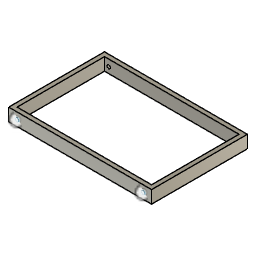
Power Supply Jig v4 (Autodesk Fusion 360 design; units mm, degrees)
Autodesk Fusion 360 part; units mm, degrees
sketch "jig" plane through (0, 0, 0) normal (0, 0, 1) x (1, 0, 0)
  line L0 (-150, 0) -> (20, 0)
  line L1 (-150, 0) -> (-150, 116)
  line L2 (-150, 116) -> (20, 116)
  line L3 (20, 116) -> (20, 0)
  line L4 (-144.988, 5.0299) -> (15.012, 5.0299)
  line L5 (-144.988, 5.0299) -> (-144.988, 111.0299)
  line L6 (15.012, 5.0299) -> (15.012, 111.0299)
  line L7 (15.012, 111.0299) -> (-144.988, 111.0299)
  dimension "d1" = 170
  dimension "d2" = 116
  dimension "d3" = 170
  dimension "d4" = 160
  dimension "d5" = 106
  dimension "d6" = 106
  constraint horizontal L0
  constraint perpendicular L0 L1
  constraint perpendicular L1 L2
  constraint perpendicular L1 L4
  constraint perpendicular L4 L5
  constraint perpendicular L4 L6
  measures "d1" distance of L0.start L0.end
  measures "d2" distance of L0.start L1.end
  measures "d3" distance of L1.end L2.end
  measures "d4" distance of L4.start L4.end
  measures "d5" distance of L4.start L5.end
  measures "d6" distance of L4.end L6.end
extrude "Extrude1" add sketch "jig" along normal blind 10
extrude "Extrude2" add 1 faces at (-91.6627, 1.6766, 10) along direction (0, 0, 1) blind 5
sketch "bolt holes" plane through (0, 0, 0) normal (0, 1, 0) x (1, 0, 0)
  circle A0 centre (10, -7) radius 2
  circle A1 centre (-140, -7) radius 2
  dimension "d11" = 4
  dimension "d12" = 4
  measures "d11" diameter of A0
  measures "d12" diameter of A1
extrude "Extrude3" cut sketch "bolt holes" along normal blind 130 contours A1
extrude "Extrude4" cut sketch "bolt holes" along normal blind 140 contours A0
extrude "Extrude5" add 1 faces at (-40.4634, 111.0299, 12.8047) along direction (0, -1, 0) blind 3
extrude "Extrude6" cut 1 faces at (-147.3309, 116, 7.3899) along direction (0, -1, 0) blind 3
extrude "Extrude7" add 1 faces at (-147.3309, 113, 7.3899) along direction (0, 1, 0) blind 1
extrude "Extrude8" cut 1 faces at (-40.4634, 108.0299, 12.8047) along direction (0, 1, 0) blind 1
named bodies: "jig"
